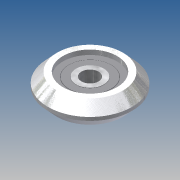
# Autodesk Inventor part: Mauro_White_Wheel
Saved by Autodesk Inventor 2015 SP1 (Build 190203100, 203)
## iProperties
Created: 2015-03-04
Part Number: Mauro_White_Wheel
Material: Generisch
Document SubType Name: Modeling
Designer: Marc
Density: 1 g/cm^3
Appearance: Vorgabe
Author: Marc
Autodesk Inventor part; units mm, degrees
ref_plane "YZ Plane" through (0, 0, 0) normal (1, 0, 0) x (0, 1, 0)
ref_plane "XZ Plane" through (0, 0, 0) normal (0, 1, 0) x (-1, 0, 0)
ref_plane "XY Plane" through (0, 0, 0) normal (0, 0, 1) x (1, 0, 0)
sketch "Skizze1" plane through (0, 0, 0) normal (0, 0, 1) x (1, 0, 0)
  circle A0 centre (0, 0) radius 3
  circle A1 centre (0, 0) radius 14.725
  dimension "d0" = 6
  dimension "d1" = 29.45
  constraints: 2 centre point, 2 coincident
  measures "d0" diameter of A0
  measures "d1" diameter of A1
extrude "Extrusion1" add sketch "Skizze1" along normal mid plane 8
sketch "Skizze2" plane through (0, 0, 4) normal (0, 0, 1) x (1, 0, 0)
  circle A0 centre (0, 0) radius 3 projected
  circle A1 centre (0, 0) radius 14.725 projected
  circle A2 centre (0, 0) radius 4.85
  circle A3 centre (0, 0) radius 4.9
  circle A4 centre (0, 0) radius 7.325
  circle A5 centre (0, 0) radius 9.5
  circle A6 centre (0, 0) radius 7.45
  dimension "d4" = 9.7
  dimension "d5" = 9.8
  dimension "d6" = 14.65
  dimension "d7" = 19
  dimension "d16" = 14.9
  constraints: 5 centre point, 5 coincident
  measures "d4" diameter of A2
  measures "d5" diameter of A3
  measures "d6" diameter of A4
  measures "d7" diameter of A5
  measures "d16" diameter of A6
extrude "Extrusion2" cut sketch "Skizze2" against normal blind 1.5 contours A2
extrude "Extrusion3" cut sketch "Skizze2" against normal blind 1.6 contours A4
extrude "Extrusion4" cut sketch "Skizze2" against normal blind 1.65 contours A5 | A6
extrude "Extrusion5" cut sketch "Skizze2" against normal blind 3 contours A3
extrude "Extrusion6" cut sketch "Skizze2" against normal blind 3 contours A6
sketch "Skizze4" plane through (0, 0, -4) normal (0, 0, -1) x (-1, 0, 0)
  circle A0 centre (0, 0) radius 3 projected
  circle A1 centre (0, 0) radius 14.725 projected
  circle A2 centre (0, 0) radius 4.9 projected
  circle A3 centre (0, 0) radius 7.45 projected
  circle A4 centre (0, 0) radius 7.325 projected
  circle A5 centre (0, 0) radius 9.5 projected
  circle A6 centre (0, 0) radius 4.85 projected
extrude "Extrusion7" add sketch "Skizze4" along normal blind 3.2 contours A6
extrude "Extrusion8" cut sketch "Skizze4" against normal blind 3 contours A2
extrude "Extrusion9" cut sketch "Skizze4" against normal blind 0.6 contours A4
extrude "Extrusion10" cut sketch "Skizze4" against normal blind 3 contours A3
extrude "Extrusion11" cut sketch "Skizze4" against normal blind 0.6 contours A5
chamfer "Fase1" distance 3.175 distance2 3.4 1 edges at (-14.725, 0, -4)
chamfer "Fase2" distance 3.175 distance2 3.4 1 edges at (-14.725, 0, 4) measured on face at (12.7487, -1.9325, 4)
